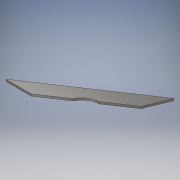
# Autodesk Inventor part: gusset
Saved by Autodesk Inventor 2018 (Build 220112000, 112)
## iProperties
Created: 2018-01-14
Part Number: gusset
Material: Stainless Steel
Document SubType Name: Modeling
Designer: prakh
Density: 8 g/cm^3
Appearance: Semi-Polished
Author: prakh
Autodesk Inventor part; units mm, degrees
ref_plane "YZ Plane" through (0, 0, 0) normal (1, 0, 0) x (0, 1, 0)
ref_plane "XZ Plane" through (0, 0, 0) normal (0, 1, 0) x (-1, 0, 0)
ref_plane "XY Plane" through (0, 0, 0) normal (0, 0, 1) x (1, 0, 0)
sketch "Sketch1" plane through (0, 0, 0) normal (0, 1, 0) x (-1, 0, 0)
  circle A0 centre (0, 0) radius 19.812
  line L0 (82.55, 0) -> (44.45, 0)
  line L1 (-16.8884, -41.1167) -> (-31.3641, -76.3597)
  line L2 (-31.3641, -76.3597) -> (82.55, 0)
  line L3 (82.55, 0) -> (101.496, 12.7)
  line L4 (101.496, 12.7) -> (63.396, 12.7)
  line L5 (63.396, 12.7) -> (44.45, 0)
  line L6 (-16.8884, -41.1167) -> (-35.8343, -53.8167)
  line L7 (-35.8343, -53.8167) -> (-50.3101, -89.0597)
  line L8 (-50.3101, -89.0597) -> (-31.3641, -76.3597)
  arc A1 (1.9176, -28.5106) -> (25.644, -12.6062) centre (0, 0) ccw
  line L9 (44.45, 0) -> (25.644, -12.6062)
  line L10 (1.9176, -28.5106) -> (-16.8884, -41.1167)
  dimension "d0" = 112.33
  dimension "d2" = 39.624
  dimension "d3" = 44.45
  dimension "d4" = 44.45
  dimension "d5" = 38.1
  dimension "d6" = 38.1
  dimension "d7" = 112.33
  dimension "d10" = 12.7
  dimension "d12" = 12.7
  dimension "d13" = 28.575
  constraints: 22 end point, 6 collinear, 2 centre point, 2 parallel, 2 point on circle, 1 coincident, 1 concentric, 1 horizontal, 1 horizontal alignment
  measures "d0" angle of L1 L0
  measures "d2" diameter of A0
  measures "d3" distance of point (0, 0) L0.end
  measures "d4" distance of L1.start point (0, 0)
  measures "d5" distance of L1.start L1.end
  measures "d6" distance of L0.start L0.end
  measures "d10" distance between parallel lines of L7 L1
  measures "d12" distance between parallel lines of L4 L0
  measures "d13" radius of A1
extrude "Extrusion1" add sketch "Sketch1" along normal blind 3.175 contours L2 L1 L10 A1 L9 L0 | L0 L5 L4 L3 | L8 L7 L6 L1
equation "\"d4\" = d3"
equation "\"d7\" = d0"
body "Solid1"
